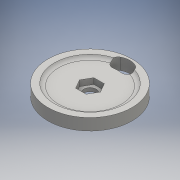
# Autodesk Inventor part: rotor
Saved by Autodesk Inventor 2016 (Build 200138000, 138)
## iProperties
Created: 2016-04-19
Part Number: rotor
Material: Generic
Document SubType Name: Modeling
Designer: Administrator
Density: 1 g/cm^3
Appearance: Default
Author: Administrator
Autodesk Inventor part; units mm, degrees
ref_plane "YZ Plane" through (0, 0, 0) normal (1, 0, 0) x (0, 1, 0)
ref_plane "XZ Plane" through (0, 0, 0) normal (0, 1, 0) x (-1, 0, 0)
ref_plane "XY Plane" through (0, 0, 0) normal (0, 0, 1) x (1, 0, 0)
sketch "Sketch1" plane through (0, 0, 0) normal (0, 0, 1) x (1, 0, 0)
  circle A0 centre (0, 0) radius 2.6757
  arc A1 (-3.2018, 16.2488) -> (-1.5837, 11.5915) centre (-2, 14.0566) ccw
  arc A2 (3.2018, 16.2488) -> (-3.2018, 16.2488) centre (0, 10.4085) ccw
  arc A3 (1.5837, 11.5915) -> (3.2018, 16.2488) centre (2, 14.0566) ccw
  arc A4 (1.5837, 11.5915) -> (-1.5837, 11.5915) centre (0, 2.2125) ccw
  circle A5 centre (0, 0) radius 18
  line L0 (-25.2, 0) -> (25.2, 0) projected
  line L1 (0, -25.2) -> (0, 25.2) projected
  dimension "d0" = 36
  dimension "d3" = 5.3514
  dimension "d10" = 4
  dimension "d11" = 2.5
  constraints: 8 point on circle, 6 centre point, 4 tangent, 1 equal radius, 1 symmetric about line
  measures "d0" diameter of A5
  measures "d3" diameter of A0
  measures "d10" distance of A3.centre A1.centre
  measures "d11" radius of A3
extrude "Extrusion1" add sketch "Sketch1" along normal blind 5 contours L0 A5 L1 A0 | A0 L1 A4 A3 A2 A5 L0 | A0 L0 A5 L1 A2 A1 A4 | L1 A5 L0 A0
sketch "Sketch2" plane through (0, 0, 5) normal (0, 0, 1) x (1, 0, 0)
  arc A0 (3.2018, 16.2488) -> (-3.2018, 16.2488) centre (0, 10.4085) ccw projected
  arc A1 (1.5837, 11.5915) -> (3.2018, 16.2488) centre (2, 14.0566) ccw projected
  arc A2 (1.5837, 11.5915) -> (-1.5837, 11.5915) centre (0, 2.2125) ccw projected
  arc A3 (-3.2018, 16.2488) -> (-1.5837, 11.5915) centre (-2, 14.0566) ccw projected
  circle A4 centre (0, 0) radius 2.6757 projected
  circle A5 centre (0, 0) radius 18 projected
  line L0 (2.25, -3.8971) -> (-2.25, -3.8971)
  line L1 (-2.25, -3.8971) -> (-4.5, 0)
  line L2 (-4.5, 0) -> (-2.25, 3.8971)
  line L3 (-2.25, 3.8971) -> (2.25, 3.8971)
  line L4 (2.25, 3.8971) -> (4.5, 0)
  line L5 (4.5, 0) -> (2.25, -3.8971)
  circle A6 centre (0, 0) radius 4.5 construction
  dimension "d4" = 9
  constraints: 12 end point, 2 coincident, 1 horizontal, 16 other
extrude "Extrusion2" cut sketch "Sketch2" against normal blind 3.5 contours L0 L1 L2 L3 L4 L5
sketch "Sketch3" plane through (0, 0, 5) normal (0, 0, 1) x (1, 0, 0)
  circle A0 centre (0, 0) radius 18 projected
  circle A1 centre (0, 0) radius 15.2203
  constraints: 1 centre point
extrude "Extrusion3" cut sketch "Sketch3" against normal blind 1 contours A1
fillet "Fillet1" radius 2 1 edges at (0, -15.2203, 4)
body "Solid1"
